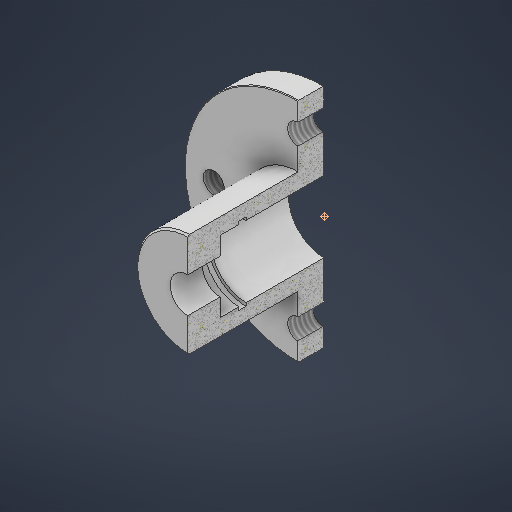
# Autodesk Inventor part: BearingSuport
Saved by Autodesk Inventor 2025.4 (Build 294407000, 407)
## iProperties
Created: 2026-05-29
Part Number: BearingSuport
Material: Generic
Document SubType Name: Modeling
Designer: VuQuan
Density: 1 g/cm^3
Appearance: Default
Author: VuQuan
Autodesk Inventor part; units mm, degrees
ref_plane "YZ Plane" through (0, 0, 0) normal (1, 0, 0) x (0, 1, 0)
ref_plane "XZ Plane" through (0, 0, 0) normal (0, 1, 0) x (-1, 0, 0)
sketch "Sketch1" plane through (0, 0, 0) normal (0, 0, 1) x (1, 0, 0)
  circle A0 centre (0, 0) radius 17.5
  circle A1 centre (0, 0) radius 8
  circle A2 centre (0, 0) radius 5.5
  circle A3 centre (0, 0) radius 2.75
  circle A4 centre (0, 0) radius 13 construction
  point P0 (0, 13)
  point P1 (-13, 0)
  point P2 (0, -13)
  point P3 (13, 0)
  dimension "d10" = 26
  dimension "d0" = 35
  dimension "d1" = 16
  dimension "d2" = 11
  dimension "d3" = 5.5
  dimension "d13" = 360
  constraints: 5 coincident, 4 centre point, 2 vertical alignment, 7 other
  measures "d0" diameter of A0
  measures "d1" diameter of A1
  measures "d2" diameter of A2
  measures "d3" diameter of A3
extrude "Extrusion1" add sketch "Sketch1" along normal blind 4 contours A0 | A1 | A2
extrude "Extrusion2" add sketch "Sketch1" along normal blind 21 contours A1 | A2
extrude "Extrusion3" cut sketch "Sketch1" along normal blind 16 contours A2
hole "Hole1" at (0, -13, 0) at (13, 0, 0) at (0, 13, 0) at (-13, 0, 0) direction (0, 0, 1) diameter 3.242 end through all thread size "M4x0.7" class "6H" standard "ISO Metric profile"
ref_plane "Work Plane1" through (0, 0, 13.1) normal (0, 0, 1) x (1, 0, 0)
sketch "Sketch2" plane through (0, 0, 13.1) normal (0, 0, 1) x (1, 0, 0)
  circle A0 centre (0, 0) radius 6
  dimension "d23" = 12
  constraints: 1 centre point, 1 coincident
  measures "d23" diameter of A0
extrude "Extrusion4" cut sketch "Sketch2" against normal blind 1.1
chamfer "Chamfer1" distance 0.25 angle 45 1 edges at (-8, 0, 21)
chamfer "Chamfer2" distance 0.1 angle 45 6 edges at (-17.5, 0, 4) (-17.5, 0, 0) (-13, -1.621, 0) (0, -14.621, 0) (0, 11.379, 0) (13, -1.621, 0)
body "Solid1"
